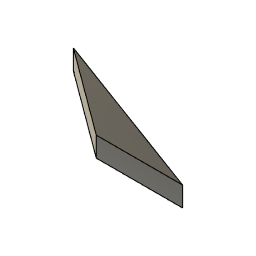
UglicZaDrzanjeKamerePodIdealnimUglom v2 (Autodesk Fusion 360 design; units mm, degrees)
Autodesk Fusion 360 part; units mm, degrees
sketch "Sketch1" plane through (0, 0, 0) normal (0, 0, 1) x (1, 0, 0)
  line L0 (51.784, 14.7352) -> (82.154, 14.7352)
  line L1 (51.784, 14.7352) -> (21.1837, 37.2656)
  line L2 (21.1837, 37.2656) -> (82.154, 14.7352)
  dimension "d1" = 30.37
  dimension "d2" = 38
  dimension "d3" = 65
  constraint horizontal L0
  measures "d1" distance of L0.start L0.end
  measures "d2" distance of L0.start L1.end
  measures "d3" distance of L0.end L1.end
extrude "Extrude1" add sketch "Sketch1" along normal blind 7
